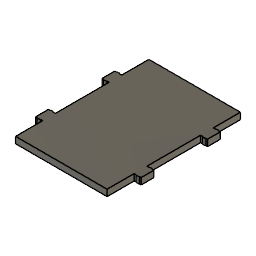
Support - Servo Support FINAL (Autodesk Fusion 360 design; units mm, degrees)
description: STEP AP242 Edition 2
part number: Servo Support
Autodesk Fusion 360 part; units mm, degrees
sketch "Sketch1" plane through (0, 0, 3.2) normal (0, 0, 1) x (-1, 0, 0)
  spline S0 degree 3 poles (18.6, -12.37) (18.6, -12.3617) (18.5987, -12.3535) (18.5936, -12.337) (18.5898, -12.3289) (18.5742, -12.3033) (18.5585, -12.2876) (18.5045, -12.2441) (18.4495, -12.2163) (18.2418, -12.1471) (18.0459, -12.12) (17.6541, -12.12) (17.4582, -12.1471) (17.2505, -12.2163) (17.1955, -12.2441) (17.1415, -12.2876) (17.1258, -12.3033) (17.1102, -12.3289) (17.1064, -12.337) (17.1013, -12.3535) (17.1, -12.3617) (17.1, -12.37) knots 0 0 0 0 0.002502 0.002502 0.005177 0.005177 0.01148 0.01148 0.02594 0.02594 0.054889 0.054889 0.083839 0.083839 0.098299 0.098299 0.104601 0.104601 0.107277 0.107277 0.109779 0.109779 0.109779 0.109779
  line L0 (17.1, -12.37) -> (16.15, -12.37)
  line L1 (16.15, -12.37) -> (16.15, 12.37)
  line L2 (16.15, 12.37) -> (17.1, 12.37)
  spline S1 degree 3 poles (17.1, 12.37) (17.1, 12.3617) (17.1013, 12.3535) (17.1064, 12.337) (17.1102, 12.3289) (17.1258, 12.3033) (17.1415, 12.2876) (17.1955, 12.2441) (17.2505, 12.2163) (17.4582, 12.1471) (17.6541, 12.12) (18.0459, 12.12) (18.2418, 12.1471) (18.4495, 12.2163) (18.5045, 12.2441) (18.5585, 12.2876) (18.5742, 12.3033) (18.5898, 12.3289) (18.5936, 12.337) (18.5987, 12.3535) (18.6, 12.3617) (18.6, 12.37) knots 0 0 0 0 0.002502 0.002502 0.005177 0.005177 0.01148 0.01148 0.02594 0.02594 0.054889 0.054889 0.083839 0.083839 0.098299 0.098299 0.104601 0.104601 0.107277 0.107277 0.109779 0.109779 0.109779 0.109779
  line L3 (18.6, 12.37) -> (19.35, 12.37)
  line L4 (19.35, 12.37) -> (19.35, 18.27)
  line L5 (19.35, 18.27) -> (18.6, 18.27)
  spline S2 degree 3 poles (18.6, 18.27) (18.6, 18.2783) (18.5987, 18.2865) (18.5936, 18.303) (18.5898, 18.3111) (18.5742, 18.3367) (18.5585, 18.3524) (18.5045, 18.3959) (18.4495, 18.4237) (18.2418, 18.4929) (18.0459, 18.52) (17.6541, 18.52) (17.4582, 18.4929) (17.2505, 18.4237) (17.1955, 18.3959) (17.1415, 18.3524) (17.1258, 18.3367) (17.1102, 18.3111) (17.1064, 18.303) (17.1013, 18.2865) (17.1, 18.2783) (17.1, 18.27) knots 0 0 0 0 0.002502 0.002502 0.005177 0.005177 0.01148 0.01148 0.02594 0.02594 0.054889 0.054889 0.083839 0.083839 0.098299 0.098299 0.104601 0.104601 0.107277 0.107277 0.109779 0.109779 0.109779 0.109779
  line L6 (17.1, 18.27) -> (16.15, 18.27)
  line L7 (16.15, 18.27) -> (16.15, 30.8)
  line L8 (16.15, 30.8) -> (-6.15, 30.8)
  line L9 (-6.15, 30.8) -> (-6.15, 18.27)
  line L10 (-6.15, 18.27) -> (-7.1, 18.27)
  spline S3 degree 3 poles (-7.1, 18.27) (-7.1, 18.2783) (-7.1013, 18.2865) (-7.1064, 18.303) (-7.1102, 18.3111) (-7.1258, 18.3367) (-7.1415, 18.3524) (-7.1955, 18.3959) (-7.2505, 18.4237) (-7.4582, 18.4929) (-7.6541, 18.52) (-8.0459, 18.52) (-8.2418, 18.4929) (-8.4495, 18.4237) (-8.5045, 18.3959) (-8.5585, 18.3524) (-8.5742, 18.3367) (-8.5898, 18.3111) (-8.5936, 18.303) (-8.5987, 18.2865) (-8.6, 18.2783) (-8.6, 18.27) knots 0 0 0 0 0.002502 0.002502 0.005177 0.005177 0.01148 0.01148 0.02594 0.02594 0.054889 0.054889 0.083839 0.083839 0.098299 0.098299 0.104601 0.104601 0.107277 0.107277 0.109779 0.109779 0.109779 0.109779
  line L11 (-8.6, 18.27) -> (-9.35, 18.27)
  line L12 (-9.35, 18.27) -> (-9.35, 12.37)
  line L13 (-9.35, 12.37) -> (-8.6, 12.37)
  spline S4 degree 3 poles (-8.6, 12.37) (-8.6, 12.3617) (-8.5987, 12.3535) (-8.5936, 12.337) (-8.5898, 12.3289) (-8.5742, 12.3033) (-8.5585, 12.2876) (-8.5045, 12.2441) (-8.4495, 12.2163) (-8.2418, 12.1471) (-8.0459, 12.12) (-7.6541, 12.12) (-7.4582, 12.1471) (-7.2505, 12.2163) (-7.1955, 12.2441) (-7.1415, 12.2876) (-7.1258, 12.3033) (-7.1102, 12.3289) (-7.1064, 12.337) (-7.1013, 12.3535) (-7.1, 12.3617) (-7.1, 12.37) knots 0 0 0 0 0.002502 0.002502 0.005177 0.005177 0.01148 0.01148 0.02594 0.02594 0.054889 0.054889 0.083839 0.083839 0.098299 0.098299 0.104601 0.104601 0.107277 0.107277 0.109779 0.109779 0.109779 0.109779
  line L14 (-7.1, 12.37) -> (-6.15, 12.37)
  line L15 (-6.15, 12.37) -> (-6.15, -12.37)
  line L16 (-6.15, -12.37) -> (-7.1, -12.37)
  spline S5 degree 3 poles (-7.1, -12.37) (-7.1, -12.3617) (-7.1013, -12.3535) (-7.1064, -12.337) (-7.1102, -12.3289) (-7.1258, -12.3033) (-7.1415, -12.2876) (-7.1955, -12.2441) (-7.2505, -12.2163) (-7.4582, -12.1471) (-7.6541, -12.12) (-8.0459, -12.12) (-8.2418, -12.1471) (-8.4495, -12.2163) (-8.5045, -12.2441) (-8.5585, -12.2876) (-8.5742, -12.3033) (-8.5898, -12.3289) (-8.5936, -12.337) (-8.5987, -12.3535) (-8.6, -12.3617) (-8.6, -12.37) knots 0 0 0 0 0.002502 0.002502 0.005177 0.005177 0.01148 0.01148 0.02594 0.02594 0.054889 0.054889 0.083839 0.083839 0.098299 0.098299 0.104601 0.104601 0.107277 0.107277 0.109779 0.109779 0.109779 0.109779
  line L17 (-8.6, -12.37) -> (-9.35, -12.37)
  line L18 (-9.35, -12.37) -> (-9.35, -18.27)
  line L19 (-9.35, -18.27) -> (-8.6, -18.27)
  spline S6 degree 3 poles (-8.6, -18.27) (-8.6, -18.2783) (-8.5987, -18.2865) (-8.5936, -18.303) (-8.5898, -18.3111) (-8.5742, -18.3367) (-8.5585, -18.3524) (-8.5045, -18.3959) (-8.4495, -18.4237) (-8.2418, -18.4929) (-8.0459, -18.52) (-7.6541, -18.52) (-7.4582, -18.4929) (-7.2505, -18.4237) (-7.1955, -18.3959) (-7.1415, -18.3524) (-7.1258, -18.3367) (-7.1102, -18.3111) (-7.1064, -18.303) (-7.1013, -18.2865) (-7.1, -18.2783) (-7.1, -18.27) knots 0 0 0 0 0.002502 0.002502 0.005177 0.005177 0.01148 0.01148 0.02594 0.02594 0.054889 0.054889 0.083839 0.083839 0.098299 0.098299 0.104601 0.104601 0.107277 0.107277 0.109779 0.109779 0.109779 0.109779
  line L20 (-7.1, -18.27) -> (-6.15, -18.27)
  line L21 (-6.15, -18.27) -> (-6.15, -30.8)
  line L22 (-6.15, -30.8) -> (16.15, -30.8)
  line L23 (16.15, -30.8) -> (16.15, -18.27)
  line L24 (16.15, -18.27) -> (17.1, -18.27)
  spline S7 degree 3 poles (17.1, -18.27) (17.1, -18.2783) (17.1013, -18.2865) (17.1064, -18.303) (17.1102, -18.3111) (17.1258, -18.3367) (17.1415, -18.3524) (17.1955, -18.3959) (17.2505, -18.4237) (17.4582, -18.4929) (17.6541, -18.52) (18.0459, -18.52) (18.2418, -18.4929) (18.4495, -18.4237) (18.5045, -18.3959) (18.5585, -18.3524) (18.5742, -18.3367) (18.5898, -18.3111) (18.5936, -18.303) (18.5987, -18.2865) (18.6, -18.2783) (18.6, -18.27) knots 0 0 0 0 0.002502 0.002502 0.005177 0.005177 0.01148 0.01148 0.02594 0.02594 0.054889 0.054889 0.083839 0.083839 0.098299 0.098299 0.104601 0.104601 0.107277 0.107277 0.109779 0.109779 0.109779 0.109779
  line L25 (18.6, -18.27) -> (19.35, -18.27)
  line L26 (19.35, -18.27) -> (19.35, -12.37)
  line L27 (19.35, -12.37) -> (18.6, -12.37)
  line L28 (-7.1, -12.37) -> (-7.1, -12.3617) construction
  line L29 (-7.1, -12.3617) -> (-7.1013, -12.3535) construction
  line L30 (-7.1013, -12.3535) -> (-7.1064, -12.337) construction
  line L31 (-7.1064, -12.337) -> (-7.1102, -12.3289) construction
  line L32 (-7.1102, -12.3289) -> (-7.1258, -12.3033) construction
  line L33 (-7.1258, -12.3033) -> (-7.1415, -12.2876) construction
  line L34 (-7.1415, -12.2876) -> (-7.1955, -12.2441) construction
  line L35 (-7.1955, -12.2441) -> (-7.2505, -12.2163) construction
  line L36 (-7.2505, -12.2163) -> (-7.4582, -12.1471) construction
  line L37 (-7.4582, -12.1471) -> (-7.6541, -12.12) construction
  line L38 (-7.6541, -12.12) -> (-8.0459, -12.12) construction
  line L39 (-8.0459, -12.12) -> (-8.2418, -12.1471) construction
  line L40 (-8.2418, -12.1471) -> (-8.4495, -12.2163) construction
  line L41 (-8.4495, -12.2163) -> (-8.5045, -12.2441) construction
  line L42 (-8.5045, -12.2441) -> (-8.5585, -12.2876) construction
  line L43 (-8.5585, -12.2876) -> (-8.5742, -12.3033) construction
  line L44 (-8.5742, -12.3033) -> (-8.5898, -12.3289) construction
  line L45 (-8.5898, -12.3289) -> (-8.5936, -12.337) construction
  line L46 (-8.5936, -12.337) -> (-8.5987, -12.3535) construction
  line L47 (-8.5987, -12.3535) -> (-8.6, -12.3617) construction
  line L48 (-8.6, -12.3617) -> (-8.6, -12.37) construction
  line L49 (18.6, 18.27) -> (18.6, 18.2783) construction
  line L50 (18.6, 18.2783) -> (18.5987, 18.2865) construction
  line L51 (18.5987, 18.2865) -> (18.5936, 18.303) construction
  line L52 (18.5936, 18.303) -> (18.5898, 18.3111) construction
  line L53 (18.5898, 18.3111) -> (18.5742, 18.3367) construction
  line L54 (18.5742, 18.3367) -> (18.5585, 18.3524) construction
  line L55 (18.5585, 18.3524) -> (18.5045, 18.3959) construction
  line L56 (18.5045, 18.3959) -> (18.4495, 18.4237) construction
  line L57 (18.4495, 18.4237) -> (18.2418, 18.4929) construction
  line L58 (18.2418, 18.4929) -> (18.0459, 18.52) construction
  line L59 (18.0459, 18.52) -> (17.6541, 18.52) construction
  line L60 (17.6541, 18.52) -> (17.4582, 18.4929) construction
  line L61 (17.4582, 18.4929) -> (17.2505, 18.4237) construction
  line L62 (17.2505, 18.4237) -> (17.1955, 18.3959) construction
  line L63 (17.1955, 18.3959) -> (17.1415, 18.3524) construction
  line L64 (17.1415, 18.3524) -> (17.1258, 18.3367) construction
  line L65 (17.1258, 18.3367) -> (17.1102, 18.3111) construction
  line L66 (17.1102, 18.3111) -> (17.1064, 18.303) construction
  line L67 (17.1064, 18.303) -> (17.1013, 18.2865) construction
  line L68 (17.1013, 18.2865) -> (17.1, 18.2783) construction
  line L69 (17.1, 18.2783) -> (17.1, 18.27) construction
  line L70 (17.1, -18.27) -> (17.1, -18.2783) construction
  line L71 (17.1, -18.2783) -> (17.1013, -18.2865) construction
  line L72 (17.1013, -18.2865) -> (17.1064, -18.303) construction
  line L73 (17.1064, -18.303) -> (17.1102, -18.3111) construction
  line L74 (17.1102, -18.3111) -> (17.1258, -18.3367) construction
  line L75 (17.1258, -18.3367) -> (17.1415, -18.3524) construction
  line L76 (17.1415, -18.3524) -> (17.1955, -18.3959) construction
  line L77 (17.1955, -18.3959) -> (17.2505, -18.4237) construction
  line L78 (17.2505, -18.4237) -> (17.4582, -18.4929) construction
  line L79 (17.4582, -18.4929) -> (17.6541, -18.52) construction
  line L80 (17.6541, -18.52) -> (18.0459, -18.52) construction
  line L81 (18.0459, -18.52) -> (18.2418, -18.4929) construction
  line L82 (18.2418, -18.4929) -> (18.4495, -18.4237) construction
  line L83 (18.4495, -18.4237) -> (18.5045, -18.3959) construction
  line L84 (18.5045, -18.3959) -> (18.5585, -18.3524) construction
  line L85 (18.5585, -18.3524) -> (18.5742, -18.3367) construction
  line L86 (18.5742, -18.3367) -> (18.5898, -18.3111) construction
  line L87 (18.5898, -18.3111) -> (18.5936, -18.303) construction
  line L88 (18.5936, -18.303) -> (18.5987, -18.2865) construction
  line L89 (18.5987, -18.2865) -> (18.6, -18.2783) construction
  line L90 (18.6, -18.2783) -> (18.6, -18.27) construction
  line L91 (-8.6, 12.37) -> (-8.6, 12.3617) construction
  line L92 (-8.6, 12.3617) -> (-8.5987, 12.3535) construction
  line L93 (-8.5987, 12.3535) -> (-8.5936, 12.337) construction
  line L94 (-8.5936, 12.337) -> (-8.5898, 12.3289) construction
  line L95 (-8.5898, 12.3289) -> (-8.5742, 12.3033) construction
  line L96 (-8.5742, 12.3033) -> (-8.5585, 12.2876) construction
  line L97 (-8.5585, 12.2876) -> (-8.5045, 12.2441) construction
  line L98 (-8.5045, 12.2441) -> (-8.4495, 12.2163) construction
  line L99 (-8.4495, 12.2163) -> (-8.2418, 12.1471) construction
  line L100 (-8.2418, 12.1471) -> (-8.0459, 12.12) construction
  line L101 (-8.0459, 12.12) -> (-7.6541, 12.12) construction
  line L102 (-7.6541, 12.12) -> (-7.4582, 12.1471) construction
  line L103 (-7.4582, 12.1471) -> (-7.2505, 12.2163) construction
  line L104 (-7.2505, 12.2163) -> (-7.1955, 12.2441) construction
  line L105 (-7.1955, 12.2441) -> (-7.1415, 12.2876) construction
  line L106 (-7.1415, 12.2876) -> (-7.1258, 12.3033) construction
  line L107 (-7.1258, 12.3033) -> (-7.1102, 12.3289) construction
  line L108 (-7.1102, 12.3289) -> (-7.1064, 12.337) construction
  line L109 (-7.1064, 12.337) -> (-7.1013, 12.3535) construction
  line L110 (-7.1013, 12.3535) -> (-7.1, 12.3617) construction
  line L111 (-7.1, 12.3617) -> (-7.1, 12.37) construction
  line L112 (17.1, 12.37) -> (17.1, 12.3617) construction
  line L113 (17.1, 12.3617) -> (17.1013, 12.3535) construction
  line L114 (17.1013, 12.3535) -> (17.1064, 12.337) construction
  line L115 (17.1064, 12.337) -> (17.1102, 12.3289) construction
  line L116 (17.1102, 12.3289) -> (17.1258, 12.3033) construction
  line L117 (17.1258, 12.3033) -> (17.1415, 12.2876) construction
  line L118 (17.1415, 12.2876) -> (17.1955, 12.2441) construction
  line L119 (17.1955, 12.2441) -> (17.2505, 12.2163) construction
  line L120 (17.2505, 12.2163) -> (17.4582, 12.1471) construction
  line L121 (17.4582, 12.1471) -> (17.6541, 12.12) construction
  line L122 (17.6541, 12.12) -> (18.0459, 12.12) construction
  line L123 (18.0459, 12.12) -> (18.2418, 12.1471) construction
  line L124 (18.2418, 12.1471) -> (18.4495, 12.2163) construction
  line L125 (18.4495, 12.2163) -> (18.5045, 12.2441) construction
  line L126 (18.5045, 12.2441) -> (18.5585, 12.2876) construction
  line L127 (18.5585, 12.2876) -> (18.5742, 12.3033) construction
  line L128 (18.5742, 12.3033) -> (18.5898, 12.3289) construction
  line L129 (18.5898, 12.3289) -> (18.5936, 12.337) construction
  line L130 (18.5936, 12.337) -> (18.5987, 12.3535) construction
  line L131 (18.5987, 12.3535) -> (18.6, 12.3617) construction
  line L132 (18.6, 12.3617) -> (18.6, 12.37) construction
  line L133 (18.6, -12.37) -> (18.6, -12.3617) construction
  line L134 (18.6, -12.3617) -> (18.5987, -12.3535) construction
  line L135 (18.5987, -12.3535) -> (18.5936, -12.337) construction
  line L136 (18.5936, -12.337) -> (18.5898, -12.3289) construction
  line L137 (18.5898, -12.3289) -> (18.5742, -12.3033) construction
  line L138 (18.5742, -12.3033) -> (18.5585, -12.2876) construction
  line L139 (18.5585, -12.2876) -> (18.5045, -12.2441) construction
  line L140 (18.5045, -12.2441) -> (18.4495, -12.2163) construction
  line L141 (18.4495, -12.2163) -> (18.2418, -12.1471) construction
  line L142 (18.2418, -12.1471) -> (18.0459, -12.12) construction
  line L143 (18.0459, -12.12) -> (17.6541, -12.12) construction
  line L144 (17.6541, -12.12) -> (17.4582, -12.1471) construction
  line L145 (17.4582, -12.1471) -> (17.2505, -12.2163) construction
  line L146 (17.2505, -12.2163) -> (17.1955, -12.2441) construction
  line L147 (17.1955, -12.2441) -> (17.1415, -12.2876) construction
  line L148 (17.1415, -12.2876) -> (17.1258, -12.3033) construction
  line L149 (17.1258, -12.3033) -> (17.1102, -12.3289) construction
  line L150 (17.1102, -12.3289) -> (17.1064, -12.337) construction
  line L151 (17.1064, -12.337) -> (17.1013, -12.3535) construction
  line L152 (17.1013, -12.3535) -> (17.1, -12.3617) construction
  line L153 (17.1, -12.3617) -> (17.1, -12.37) construction
  line L154 (-7.1, 18.27) -> (-7.1, 18.2783) construction
  line L155 (-7.1, 18.2783) -> (-7.1013, 18.2865) construction
  line L156 (-7.1013, 18.2865) -> (-7.1064, 18.303) construction
  line L157 (-7.1064, 18.303) -> (-7.1102, 18.3111) construction
  line L158 (-7.1102, 18.3111) -> (-7.1258, 18.3367) construction
  line L159 (-7.1258, 18.3367) -> (-7.1415, 18.3524) construction
  line L160 (-7.1415, 18.3524) -> (-7.1955, 18.3959) construction
  line L161 (-7.1955, 18.3959) -> (-7.2505, 18.4237) construction
  line L162 (-7.2505, 18.4237) -> (-7.4582, 18.4929) construction
  line L163 (-7.4582, 18.4929) -> (-7.6541, 18.52) construction
  line L164 (-7.6541, 18.52) -> (-8.0459, 18.52) construction
  line L165 (-8.0459, 18.52) -> (-8.2418, 18.4929) construction
  line L166 (-8.2418, 18.4929) -> (-8.4495, 18.4237) construction
  line L167 (-8.4495, 18.4237) -> (-8.5045, 18.3959) construction
  line L168 (-8.5045, 18.3959) -> (-8.5585, 18.3524) construction
  line L169 (-8.5585, 18.3524) -> (-8.5742, 18.3367) construction
  line L170 (-8.5742, 18.3367) -> (-8.5898, 18.3111) construction
  line L171 (-8.5898, 18.3111) -> (-8.5936, 18.303) construction
  line L172 (-8.5936, 18.303) -> (-8.5987, 18.2865) construction
  line L173 (-8.5987, 18.2865) -> (-8.6, 18.2783) construction
  line L174 (-8.6, 18.2783) -> (-8.6, 18.27) construction
  line L175 (-8.6, -18.27) -> (-8.6, -18.2783) construction
  line L176 (-8.6, -18.2783) -> (-8.5987, -18.2865) construction
  line L177 (-8.5987, -18.2865) -> (-8.5936, -18.303) construction
  line L178 (-8.5936, -18.303) -> (-8.5898, -18.3111) construction
  line L179 (-8.5898, -18.3111) -> (-8.5742, -18.3367) construction
  line L180 (-8.5742, -18.3367) -> (-8.5585, -18.3524) construction
  line L181 (-8.5585, -18.3524) -> (-8.5045, -18.3959) construction
  line L182 (-8.5045, -18.3959) -> (-8.4495, -18.4237) construction
  line L183 (-8.4495, -18.4237) -> (-8.2418, -18.4929) construction
  line L184 (-8.2418, -18.4929) -> (-8.0459, -18.52) construction
  line L185 (-8.0459, -18.52) -> (-7.6541, -18.52) construction
  line L186 (-7.6541, -18.52) -> (-7.4582, -18.4929) construction
  line L187 (-7.4582, -18.4929) -> (-7.2505, -18.4237) construction
  line L188 (-7.2505, -18.4237) -> (-7.1955, -18.3959) construction
  line L189 (-7.1955, -18.3959) -> (-7.1415, -18.3524) construction
  line L190 (-7.1415, -18.3524) -> (-7.1258, -18.3367) construction
  line L191 (-7.1258, -18.3367) -> (-7.1102, -18.3111) construction
  line L192 (-7.1102, -18.3111) -> (-7.1064, -18.303) construction
  line L193 (-7.1064, -18.303) -> (-7.1013, -18.2865) construction
  line L194 (-7.1013, -18.2865) -> (-7.1, -18.2783) construction
  line L195 (-7.1, -18.2783) -> (-7.1, -18.27) construction
extrude "Extrude1" add sketch "Sketch1" against normal blind 3
move_face "MoveFace1" to x (1, 0, 0) y (0, 1, 0) z (0, 0, 1) at (20, 0, 0) 17 faces at (6.4667, -18.27, 2.2) (6.15, -4.1233, 2.2) (9.35, -16.3033, 2.2) (9.1, 18.27, 2.2) (6.15, 22.4467, 2.2) (6.7833, 18.27, 2.2) (8.123, -12.1375, 3) (6.15, -26.6233, 2.2) (6.7833, -12.37, 2.2) (7.577, 12.1375, 3) (7.577, -18.5025, 3) (6.4667, 12.37, 2.2) (8.123, 18.5025, 3) (8.85, -18.27, 2.2) (9.1, -12.37, 2.2) (8.85, 12.37, 2.2) (9.35, 14.3367, 2.2)
